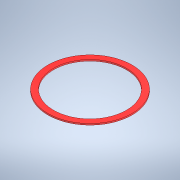
# Autodesk Inventor part: supportRingsForLargeCap
Saved by Autodesk Inventor 2021.1 (Build 251245010, 245A)
## iProperties
Created: 2020-09-25
Part Number: supportRingsForLargeCap
Material: PC/ABS Plastic
Document SubType Name: Modeling
Designer: robst
Density: 0.357273 g/cm^3
Appearance: Light Red
Author: robst
Autodesk Inventor part; units mm, degrees
ref_plane "YZ Plane" through (0, 0, 0) normal (1, 0, 0) x (0, 1, 0)
ref_plane "XZ Plane" through (0, 0, 0) normal (0, 1, 0) x (-1, 0, 0)
ref_plane "XY Plane" through (0, 0, 0) normal (0, 0, 1) x (1, 0, 0)
sketch "Sketch6" plane through (0, 0, 0) normal (0, 0, 1) x (1, 0, 0)
  line L0 (82.55, 0) -> (95.25, 0)
  line L1 (95.25, 0) -> (95.25, 3.175)
  line L2 (95.25, 3.175) -> (82.55, 3.175)
  line L3 (82.55, 3.175) -> (82.55, 0)
  line L4 (0, -0.635) -> (0, 3.81) projected
  point P0 (0, 0)
  dimension "d25" = 12.7
  dimension "d26" = 3.175
  dimension "d27" = 82.55
  constraints: 8 end point, 2 parallel, 1 horizontal, 1 perpendicular
  measures "d25" distance between parallel lines of L1 L3
  measures "d26" distance between parallel lines of L2 L0
  measures "d27" distance of L0.start point (0, 0)
revolve "Revolution3" add sketch "Sketch6" angle 360 about axis through (0, -10, 0) along (0, 1, 0)
equation "\"d25\" = glueRingWidth"
equation "\"d26\" = glueRingHeight"
equation "\"d27\" = glueRingInnerEdge"
equation "\"outsideDiameter\" = 152.4"
equation "\"thickness\" = 6.35"
equation "\"glueRingDiameter\" = 177.8"
equation "\"textRingDiameter\" = 76.2"
equation "\"textRingDepth\" = 1.27"
equation "\"glueRingRadius\" = 0.5 * glueRingDiameter"
equation "\"glueRingWidth\" = 12.7"
equation "\"glueRingHeight\" = 3.175"
equation "\"glueRingInnerEdge\" = glueRingRadius - 0.5 * glueRingWidth"
body "Solid3"
